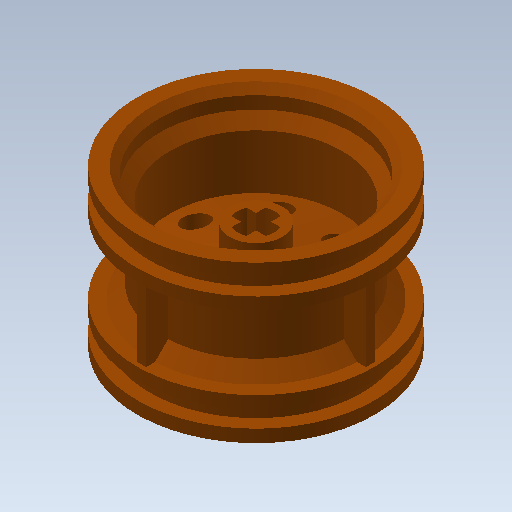
# Autodesk Inventor part: 56145_Wheel
Saved by Autodesk Inventor 2020 (Build 240168000, 168)
## iProperties
Created: 2012-09-28
Part Number: 56145_Wheel
Document SubType Name: Modeling
Designer: RChave01
Material: Genérico
Density: 1 g/cm^3
Appearance: Orange (Dark)
Author: RChave01
Autodesk Inventor part; units mm, degrees
ref_plane "YZ Plane" through (0, 0, 0) normal (1, 0, 0) x (0, 1, 0)
ref_plane "XZ Plane" through (0, 0, 0) normal (0, 1, 0) x (-1, 0, 0)
sketch "Sketch1" plane through (0, 0, 0) normal (0, 0, 1) x (1, 0, 0)
  line L0 (0, 0) -> (0, 34.5214)
  line L1 (0, 0) -> (1.1137, 0)
  line L2 (1.1137, 0) -> (1.1137, 4)
  line L3 (1.1137, 4) -> (3.3754, 4)
  line L4 (3.3754, 4) -> (3.3754, 1.2)
  line L5 (3.3754, 1.2) -> (11, -0.5899)
  line L6 (11, -0.5899) -> (11, 6.3612)
  line L7 (11, 6.3612) -> (12.35, 7.7112)
  line L8 (12.35, 7.7112) -> (12.35, 9.3)
  line L9 (12.35, 9.3) -> (13.25, 10.2)
  line L10 (13.25, 10.2) -> (15.2, 10.2)
  line L11 (15.2, 10.2) -> (15.2, 8.6)
  line L12 (15.2, 8.6) -> (13.55, 8.6)
  line L13 (13.55, 8.6) -> (13.55, 6.45)
  line L14 (13.55, 6.45) -> (15.2, 6.45)
  line L15 (15.2, 6.45) -> (15.2, 4.88)
  line L16 (15.2, 4.88) -> (13.55, 4.88)
  line L17 (13.55, 4.88) -> (11.87, 3.2)
  line L18 (11.87, 3.2) -> (11.87, -2.8)
  line L19 (11.87, -2.8) -> (13.55, -4.48)
  line L20 (13.55, -4.48) -> (15.2, -4.48)
  line L21 (15.2, -4.48) -> (15.2, -6.05)
  line L22 (15.2, -6.05) -> (13.55, -6.05)
  line L23 (13.55, -6.05) -> (13.55, -8.2)
  line L24 (13.55, -8.2) -> (15.2, -8.2)
  line L25 (15.2, -8.2) -> (15.2, -9.8)
  line L26 (15.2, -9.8) -> (13.25, -9.8)
  line L27 (13.25, -9.8) -> (12.35, -8.9)
  line L28 (12.35, -8.9) -> (12.35, -5.7513)
  line L29 (12.35, -5.7513) -> (11, -4.4013)
  line L30 (11, -4.4013) -> (11, -2.3)
  line L31 (11, -2.3) -> (5, -0.8915)
  line L32 (5, -0.8915) -> (5, -1.8)
  line L33 (5, -1.8) -> (3.7, -1.8)
  line L34 (3.7, -1.8) -> (3.7, -7.58)
  line L35 (3.7, -7.58) -> (0, -7.58)
  line L36 (0, -7.58) -> (0, 0)
  dimension "d1" = 4
  dimension "d2" = 15.2
  dimension "d3" = 12.35
  dimension "d4" = 11
  dimension "d5" = 13.25
  dimension "d6" = 45
  dimension "d7" = 45
  dimension "d8" = 9
  dimension "d9" = 6.2
  dimension "d10" = 1.6
  dimension "d12" = 1.57
  dimension "d13" = 1.57
  dimension "d14" = 1.6
  dimension "d15" = 2.15
  dimension "d16" = 2.15
  dimension "d17" = 6
  dimension "d18" = 45
  dimension "d19" = 45
  dimension "d20" = 20
  dimension "d21" = 1.65
  dimension "d22" = 1.65
  dimension "d23" = 1.65
  dimension "d24" = 13.25
  dimension "d25" = 12.35
  dimension "d26" = 11
  dimension "d27" = 7.5
  dimension "d28" = 2.22
  dimension "d29" = 8
  dimension "d30" = 3.7
  dimension "d31" = 5
  constraints: 74 end point, 30 parallel, 4 collinear, 3 perpendicular, 1 vertical, 1 other
  measures "d1" distance between parallel lines of L3 L1
  measures "d2" distance between parallel lines of L11 L36
  measures "d3" distance between parallel lines of L0 L8
  measures "d4" distance between parallel lines of L0 L6
  measures "d5" distance from line of L0 L9.end
  measures "d6" angle of L9 L10
  measures "d7" angle of L10 L7
  measures "d8" distance from line of L10 L4.end
  measures "d9" distance between parallel lines of L3 L10
  measures "d10" distance between parallel lines of L12 L10
  measures "d12" distance between parallel lines of L16 L14
  measures "d13" distance between parallel lines of L20 L22
  measures "d14" distance between parallel lines of L26 L24
  measures "d15" distance between parallel lines of L12 L14
  measures "d16" distance between parallel lines of L22 L24
  measures "d17" distance of L17.end L18.end
  measures "d18" angle of L17 L16
  measures "d19" angle of L20 L19
  measures "d20" distance between parallel lines of L26 L10
  measures "d21" distance between parallel lines of L13 L11
  measures "d22" distance from line of L16.end L15
  measures "d23" distance from line of L19.end L21
  measures "d24" distance from line of L36 L26.end
  measures "d25" distance from line of L27.end L36
  measures "d26" distance between parallel lines of L36 L30
  measures "d27" distance from line of L30.end L26
  measures "d28" distance between parallel lines of L35 L26
  measures "d29" distance between parallel lines of L33 L26
  measures "d30" distance between parallel lines of L36 L34
  measures "d31" distance between parallel lines of L36 L32
revolve "Revolution1" add sketch "Sketch1" angle 360 about axis through (0, 0, 0) along (0, 1, 0)
sketch "Sketch2" plane through (0, -7.58, 0) normal (0, -1, 0) x (1, 0, 0)
  circle A0 centre (0, 0) radius 3.7 projected
  line L0 (0, 0) -> (0, 1.7732)
  line L1 (0, 0) -> (1.2048, 0)
  line L2 (-0.96, 2.6912) -> (0.96, 2.6912)
  line L3 (0.96, -2.699) -> (-0.96, -2.699)
  line L4 (2.9937, 0.96) -> (2.9937, -0.96)
  line L5 (-2.8908, -0.96) -> (-2.8908, 0.96)
  arc A1 (2.1723, -0.96) -> (2.1723, 0.96) centre (0, 0) ccw
  arc A2 (0.96, 2.1723) -> (-0.96, 2.1723) centre (0, 0) ccw
  arc A3 (-2.1723, 0.96) -> (-2.1723, -0.96) centre (0, 0) ccw
  arc A4 (-0.96, -2.1723) -> (0.96, -2.1723) centre (0, 0) ccw
  line L6 (-0.96, -2.1723) -> (-0.96, -0.96)
  line L7 (-0.96, 0.96) -> (-0.96, 2.1723)
  line L8 (-2.1723, 0.96) -> (-0.96, 0.96)
  line L9 (0.96, 0.96) -> (2.1723, 0.96)
  line L10 (0.96, 2.1723) -> (0.96, 0.96)
  line L11 (0.96, -0.96) -> (0.96, -2.1723)
  line L12 (2.1723, -0.96) -> (0.96, -0.96)
  line L13 (-0.96, -0.96) -> (-2.1723, -0.96)
  constraints: 28 end point, 10 parallel, 8 point on circle, 5 perpendicular, 4 centre point, 3 horizontal, 1 coincident, 1 vertical
extrude "Extrusion1" cut sketch "Sketch2" against normal through all contours L12 L11 A4 L6 L13 A3 L8 L7 A2 L10 L9 A1
ref_plane "Work Plane1" through (0, -7.42, 0) normal (0, -1, 0) x (1, 0, 0)
sketch "Sketch3" plane through (0, -7.42, 0) normal (0, -1, 0) x (1, 0, 0)
  line L0 (0, 0) -> (0, 12.7754)
  circle A0 centre (0, 0) radius 12.35 projected
  line L1 (-0.85, 12.3207) -> (-1.15, 4.866)
  line L2 (0.85, 12.3207) -> (1.15, 4.866)
  circle A1 centre (0, 0) radius 5 projected
  line L3 (-1.68, 12.2352) -> (-2.0496, 4.5606)
  line L4 (1.68, 12.2352) -> (2.0496, 4.5606)
  dimension "d38" = 0.83
  dimension "d39" = 0.95
  dimension "d40" = 1.7
  dimension "d41" = 2.3
  constraints: 10 end point, 8 point on circle, 2 vertical, 2 other
  measures "d38" horizontal distance of L1.start L3.start
  measures "d39" distance of L3.end L1.end
  measures "d40" distance of L2.start L1.start
  measures "d41" distance of L2.end L1.end
extrude "Extrusion2" add sketch "Sketch3" against normal up to next contours L2 A0 L4 A1 | A1 L3 A0 L1
sketch "Sketch4" plane through (0, -7.58, 0) normal (0, -1, 0) x (1, 0, 0)
  arc A0 (0.96, 2.1723) -> (-0.96, 2.1723) centre (0, 0) ccw projected
  line L0 (-2.1723, 0.96) -> (-0.96, 0.96) projected
  circle A1 centre (0, 0) radius 3.7 projected
  line L1 (0, 0) -> (4.5386, 7.8611)
  line L2 (0, 0) -> (0, 7.372)
  circle A2 centre (3.875, 6.7117) radius 1.6
  dimension "d44" = 30
  dimension "d45" = 3.2
  dimension "d46" = 7.75
  constraints: 4 end point, 1 centre point, 1 perpendicular, 1 point on line
  measures "d44" angle of L1 L2
  measures "d45" diameter of A2
  measures "d46" distance of A2.centre A0.centre
extrude "Extrusion3" cut sketch "Sketch4" against normal through all contours A2
pattern_circular "Circular Pattern1" count 6 over 360 about axis through (0, -1.5957, 0) along (0, -1, 0) of "Extrusion2", "Extrusion3"
sketch "Sketch5" plane through (0, 0, 0) normal (1, 0, 0) x (0, 1, 0)
  line L0 (-4.48, 15.2) -> (-4.48, -15.2) projected
  line L1 (-2.8, 11.87) -> (-4.48, 13.55) projected
  line L2 (3.2, 11.87) -> (-2.8, 11.87) projected
  line L3 (4.88, 13.55) -> (3.2, 11.87) projected
  line L4 (4.88, 15.2) -> (4.88, -15.2) projected
  line L5 (-4.48, 14.67) -> (4.88, 14.67)
  line L6 (-4.48, 14.67) -> (-4.8508, 13.5618)
  line L7 (-4.8508, 13.5618) -> (-2.9729, 11.5157)
  line L8 (-2.9729, 11.5157) -> (3.5858, 11.5157)
  line L9 (3.5858, 11.5157) -> (5.4077, 13.5618)
  line L10 (5.4077, 13.5618) -> (4.88, 14.67)
  dimension "d52" = 2.8
  constraints: 12 end point, 2 perpendicular, 2 point on line
  measures "d52" distance between parallel lines of L5 L2
extrude "Extrusion4" add sketch "Sketch5" along normal mid plane 1.2
pattern_circular "Circular Pattern2" count 4 over 360 about axis through (0, 0.2, 0) along (0, -1, 0) of "Extrusion4"
equation "\"d34\" = d33"
equation "\"d33\" = 1.92"
